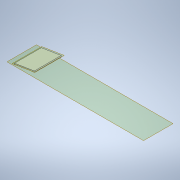
# Autodesk Inventor part: arc n°1
Saved by Autodesk Inventor 2020.2 (Build 242310000, 310)
## iProperties
Created: 2020-01-28
Part Number: arc n°1
Material: Générique
Document SubType Name: Modeling
Designer: anton
Density: 1 g/cm^3
Appearance: Par défaut
Author: anton
Autodesk Inventor part; units mm, degrees
ref_plane "YZ Plane" through (0, 0, 0) normal (1, 0, 0) x (0, 1, 0)
ref_plane "XZ Plane" through (0, 0, 0) normal (0, 1, 0) x (-1, 0, 0)
ref_plane "XY Plane" through (0, 0, 0) normal (0, 0, 1) x (1, 0, 0)
sketch "Esquisse1" plane through (0, 0, 0) normal (0, 0, 1) x (1, 0, 0)
  line L0 (-150.5839, 785.7) -> (150.5839, 785.7)
  arc A0 (150.5839, 785.7) -> (-150.5839, 785.7) centre (0, 0) ccw
  line L1 (-150.5839, 782.7) -> (150.5839, 782.7)
  line L2 (0, 797) -> (-150.5839, 797)
  arc A1 (150.5839, 782.7) -> (-150.5839, 782.7) centre (0, -3) ccw
  line L3 (-150.5839, 785.7) -> (-150.5839, 782.7)
  line L4 (150.5839, 785.7) -> (150.5839, 782.7)
  point P0 (0, 0)
  dimension "d4" = 785.7
  dimension "d8" = 3
  dimension "d9" = 14.3
  constraints: 10 end point, 5 point on circle, 3 horizontal, 2 centre point, 1 perpendicular
  measures "d4" distance from line of point (0, 0) L0
  measures "d8" distance between parallel lines of L0 L1
  measures "d9" distance between parallel lines of L1 L2
extrude "Extrusion1" add sketch "Esquisse1" along normal blind 65 contours A0 L2 A1 L0 | L0 A1 L3 | A0 L0 A1 L2 | L0 L4 A1
ref_plane "Plan de construction1" through (-150.5839, 782.7, 65) normal (0, -1, 0) x (0, 0, -1)
sketch "Esquisse2" plane through (-150.5839, 782.7, 65) normal (0, -1, 0) x (0, 0, -1)
  line L0 (65, 301.1678) -> (65, 0) projected
  line L1 (0, 0) -> (65, 0)
  line L2 (65, 0) -> (65, 48)
  line L3 (65, 48) -> (0, 48)
  line L4 (0, 48) -> (0, 0)
  line L5 (0, 48) -> (65, 48)
  line L6 (65, 48) -> (65, 301.1678)
  line L7 (65, 301.1678) -> (0, 301.1678)
  line L8 (0, 301.1678) -> (0, 48)
  point P0 (65, 150.5839)
  dimension "d13" = 48
  constraints: 16 end point, 4 parallel, 2 horizontal, 2 perpendicular, 1 point on line
  measures "d13" distance of L3.end L1.start
extrude "Extrusion2" cut sketch "Esquisse2" against normal through all contours L0 L3 L8 L7
ref_plane "Plan de construction2" through (-150.5839, 785.7, 0) normal (0.158303, -0.9873906, 0) x (0.9873906, 0.158303, 0)
sketch "Esquisse3" plane through (-150.5839, 785.7, 0) normal (0.158303, -0.9873906, 0) x (0.9873906, 0.158303, 0)
  line L0 (48.613, 65) -> (48.613, 0) projected
  line L1 (0, 0) -> (-0.4749, 0) projected
  line L2 (48.613, 65) -> (0, 65)
  line L3 (0, 65) -> (0, 0)
  line L4 (0, 0) -> (48.613, 0)
  line L5 (48.613, 0) -> (48.613, 65)
  point P0 (24.3065, 0)
  point P1 (48.613, 0)
  constraints: 8 end point, 2 parallel, 1 horizontal, 1 perpendicular
extrude "Extrusion3" cut sketch "Esquisse3" against normal blind 10
